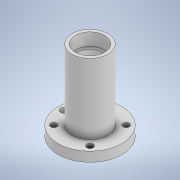
# Autodesk Inventor part: base marcador
Saved by Autodesk Inventor 2022 (Build 260153000, 153)
## iProperties
Created: 2022-08-27
Part Number: base marcador
Material: Generic
Document SubType Name: Modeling
Designer: alejo
Density: 1 g/cm^3
Appearance: Default
Author: alejo
Autodesk Inventor part; units mm, degrees
ref_plane "YZ Plane" through (0, 0, 0) normal (1, 0, 0) x (0, 1, 0)
ref_plane "XZ Plane" through (0, 0, 0) normal (0, 1, 0) x (-1, 0, 0)
ref_plane "XY Plane" through (0, 0, 0) normal (0, 0, 1) x (1, 0, 0)
sketch "Sketch1" plane through (0, 0, 0) normal (0, 1, 0) x (-1, 0, 0)
  circle A0 centre (0, 0) radius 250
  circle A1 centre (0, 0) radius 200 construction
  line L0 (0, 0) -> (0, -250) construction
  line L1 (0, 0) -> (176.7767, 176.7767) construction
  line L2 (0, 0) -> (250, 0) construction
  line L3 (176.7767, 176.7767) -> (-176.7767, -176.7767) construction
  line L4 (176.7767, -176.7767) -> (-176.7767, 176.7767) construction
  circle A2 centre (141.4214, 141.4214) radius 25
  circle A3 centre (-141.4214, 141.4214) radius 25
  circle A4 centre (-141.4214, -141.4214) radius 25
  circle A5 centre (141.4214, -141.4214) radius 25
  circle A6 centre (200, 0) radius 30
  dimension "d0" = 500
  dimension "d1" = 400
  dimension "d2" = 45
  dimension "d3" = 50
  dimension "d4" = 50
  dimension "d5" = 50
  dimension "d6" = 50
  dimension "d7" = 60
  constraints: 10 end point, 10 point on circle, 7 centre point, 6 point on line, 2 coincident, 1 equal length, 1 horizontal, 1 perpendicular, 1 vertical
  measures "d0" diameter of A0
  measures "d1" diameter of A1
  measures "d2" angle of L2 L1
  measures "d3" diameter of A2
  measures "d4" diameter of A3
  measures "d5" diameter of A4
  measures "d6" diameter of A5
  measures "d7" diameter of A6
extrude "Extrusion1" add sketch "Sketch1" along normal blind 75
sketch "Sketch2" plane through (0, 75, 0) normal (0, 1, 0) x (1, 0, 0)
  circle A0 centre (0, 0) radius 140
  circle A1 centre (0, 0) radius 92.5
  dimension "d10" = 280
  dimension "d11" = 185
  constraints: 2 centre point, 2 coincident
  measures "d10" diameter of A0
  measures "d11" diameter of A1
extrude "Extrusion2" add sketch "Sketch2" along normal blind 550
sketch "Sketch4" plane through (0, 625, 0) normal (0, 1, 0) x (1, 0, 0)
  circle A0 centre (0, 0) radius 115
  dimension "d22" = 230
  constraints: 1 centre point, 1 coincident
  measures "d22" diameter of A0
extrude "Extrusion4" cut sketch "Sketch4" against normal blind 100
body "Solid1"
